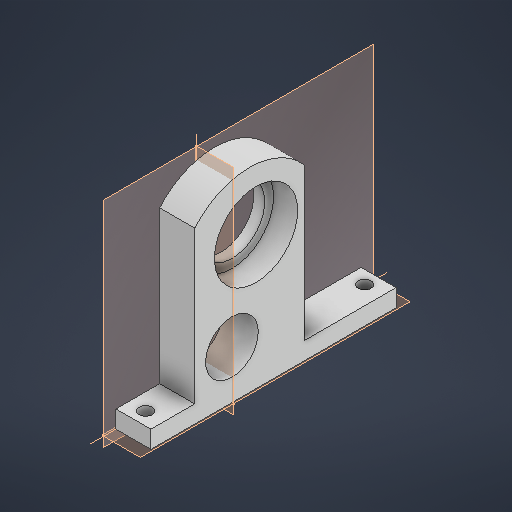
# Autodesk Inventor part: support_arriere_gauche_2
Saved by Autodesk Inventor 2027.1 (Build 311270010, 270A)
## iProperties
Created: 2026-09-15
Part Number: support_arriere_gauche_2
Material: Generic
Document SubType Name: Modeling
Designer: thiag
Density: 1 g/cm^3
Appearance: Default
Author: thiag
Autodesk Inventor part; units mm, degrees
sketch "Sketch1" plane through (0, 0, 0) normal (1, 0, 0) x (0, 1, 0)
  circle A0 centre (11, 0) radius 6
  circle A1 centre (30.5, -5.5) radius 7.5
  line L0 (0, 29.7) -> (0, -48.7) projected
  line L1 (-8.9, 0) -> (53.4, 0) projected
  line L2 (4, 18.5) -> (0, 18.5)
  line L3 (0, -37.5) -> (4, -37.5)
  line L4 (0, 18.5) -> (0, -37.5)
  line L5 (4, 18.5) -> (4, 8.5)
  line L6 (4, -37.5) -> (4, -16.5)
  line L7 (4, -16.5) -> (38.7703, -16.5)
  line L8 (38.7703, 8.5) -> (4, 8.5)
  arc A2 (38.7703, -16.5) -> (38.7703, 8.5) centre (28, -4) ccw
  point P0 (0, 0)
  dimension "d0" = 12
  dimension "d1" = 15
  dimension "d2" = 11
  dimension "d3" = 30.5
  dimension "d4" = 0
  dimension "d5" = 5.5
  dimension "d7" = 56
  dimension "d8" = 4
  dimension "d9" = 4
  dimension "d10" = 0
  dimension "d11" = 0
  dimension "d13" = 11
  dimension "d17" = 16.5
  dimension "d18" = 18.5
  dimension "d19" = 4
  dimension "d20" = 28
  dimension "d21" = 8.5
  constraints: 14 end point, 3 centre point, 2 point on circle, 2 vertical, 1 horizontal, 1 parallel, 1 perpendicular
  measures "d0" diameter of A0
  measures "d1" diameter of A1
  measures "d2" distance from line of L0 A0.centre
  measures "d3" distance from line of L0 A1.centre
  measures "d4" distance from line of L1 A0.centre
  measures "d5" distance from line of L1 A1.centre
  measures "d7" distance between parallel lines of L3 L2
  measures "d8" distance of L2.start L2.end
  measures "d9" distance of L3.start L3.end
  measures "d10" distance from line of L0 L2.end
  measures "d11" distance from line of L0 L3.start
  measures "d13" distance from line of L7 A1.centre
  measures "d17" radius of A2
  measures "d18" distance between parallel lines of L1 L2
  measures "d19" distance from line of L1 A2.centre
  measures "d20" distance from line of L0 A2.centre
  measures "d21" distance between parallel lines of L1 L8
extrude "Extrusion1" add sketch "Sketch1" along normal blind 8 contours L1 A1 A2 L7 L6 L3 L0 A0 | A0 L1 L0 L2 L5 L8 A2 A1
sketch "Sketch2" plane through (8, 0, 0) normal (1, 0, 0) x (0, 0, -1)
  circle A0 centre (5.5, 30.5) radius 9.5
  line L0 (-18.5, 0) -> (37.5, 0) projected
  line L1 (0, -8.9) -> (0, 53.4) projected
  point P0 (0, 0)
  dimension "d24" = 19
  dimension "d25" = 30.5
  dimension "d26" = 5.5
  constraints: 1 centre point
  measures "d24" diameter of A0
  measures "d25" distance from line of L0 A0.centre
  measures "d26" distance from line of L1 A0.centre
extrude "Extrusion2" cut sketch "Sketch2" against normal blind 5.5
sketch "Sketch3" plane through (0, 0, 0) normal (0, 1, 0) x (-1, 0, 0)
  circle A0 centre (-3.8, 15.5) radius 1.5
  line L0 (-8, 8.5) -> (-8, 18.5) projected
  line L1 (-9.6, 0) -> (1.6, 0) projected
  circle A1 centre (-3.8, -34.5) radius 1.5
  line L2 (-8, -37.5) -> (-8, -16.5) projected
  point P0 (0, 0)
  dimension "d29" = 3
  dimension "d30" = 4.2
  dimension "d31" = 15.5
  dimension "d32" = 3
  dimension "d33" = 4.2
  dimension "d34" = 50
  constraints: 2 centre point
  measures "d29" diameter of A0
  measures "d30" distance from line of L0 A0.centre
  measures "d31" distance from line of L1 A0.centre
  measures "d32" diameter of A1
  measures "d33" distance from line of L2 A1.centre
  measures "d34" distance of A0.centre A1.centre
extrude "Extrusion3" cut sketch "Sketch3" along normal blind 4
body "Solid1"
